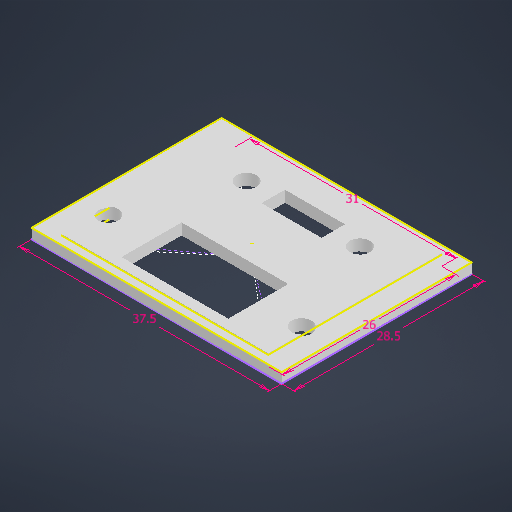
# Autodesk Inventor part: USB inner clamp plate
Saved by Autodesk Inventor 2026.2 (Build 302298010, 298A)
## iProperties
Created: 2026-04-19
Part Number: USB inner clamp plate
Material: Generic
Document SubType Name: Modeling
Designer: Graeme
Density: 1 g/cm^3
Appearance: Default
Author: Graeme
## iProperties of the stored document USB inner clamp plate_3DPrint.ipt
Created: 2026-09-30
Part Number: USB inner clamp plate_3DPrint
Material: Generic
Document SubType Name: Modeling
Designer: Graeme
Density: 1 g/cm^3
Appearance: Default
Author: Graeme
Autodesk Inventor part; units mm, degrees
ref_plane "YZ Plane" through (0, 0, 0) normal (1, 0, 0) x (0, 1, 0)
ref_plane "XZ Plane" through (0, 0, 0) normal (0, 1, 0) x (-1, 0, 0)
ref_plane "XY Plane" through (0, 0, 0) normal (0, 0, 1) x (1, 0, 0)
sketch "Sketch1" plane through (0, 0, 0) normal (0, 1, 0) x (-1, 0, 0)
  line L0 (15.5, 13) -> (-15.5, 13)
  line L1 (-15.5, 13) -> (-15.5, -13)
  line L2 (-15.5, -13) -> (15.5, -13)
  line L3 (15.5, -13) -> (15.5, 13)
  line L4 (15.5, 13) -> (-15.5, -13) construction
  line L5 (-15.5, 13) -> (15.5, -13) construction
  line L6 (18.75, -14.25) -> (-18.75, -14.25)
  line L7 (-18.75, -14.25) -> (-18.75, 14.25)
  line L8 (-18.75, 14.25) -> (18.75, 14.25)
  line L9 (18.75, 14.25) -> (18.75, -14.25)
  line L10 (18.75, -14.25) -> (-18.75, 14.25) construction
  line L11 (-18.75, -14.25) -> (18.75, 14.25) construction
  point P0 (0, 0)
  dimension "d0" = 31
  dimension "d1" = 26
  dimension "d16" = 37.5
  dimension "d17" = 28.5
  constraints: 24 end point, 4 parallel, 2 horizontal, 2 midpoint, 2 perpendicular
  measures "d0" distance of L2.end L1.end
  measures "d1" distance of L1.end L0.end
  measures "d16" distance of L7.end L8.end
  measures "d17" distance of L6.end L7.end
extrude "Extrusion2" add sketch "Sketch1" along normal blind 1.5 contours L3 L2 L1 L0 | L6 L7 L8 L9
sketch "Sketch2" plane through (0, 1.5, 0) normal (0, 1, 0) x (1, 0, 0)
  line L0 (15.5, 13) -> (-15.5, 13) projected
  line L1 (-15.5, -13) -> (15.5, -13) projected
  line L2 (-18.75, -14.25) -> (18.75, -14.25) projected
  line L3 (18.75, -14.25) -> (18.75, 14.25) projected
  line L4 (18.75, 14.25) -> (-18.75, 14.25) projected
  line L5 (-18.75, 14.25) -> (-18.75, -14.25) projected
  line L6 (15.5, -13) -> (15.5, 13) projected
  line L7 (-15.5, 13) -> (-15.5, -13) projected
  point P0 (0, 0)
extrude "Extrusion4" add sketch "Sketch2" along normal blind 0.2 contours L6 L1 L7 L0
sketch "Sketch3" plane through (0, 1.7, 0) normal (0, 1, 0) x (1, 0, 0)
  circle A0 centre (-14.5, -7) radius 1.5
  circle A1 centre (14.5, -7) radius 1.5
  circle A2 centre (-8.5, 7.75) radius 1.5
  circle A3 centre (8.5, 7.75) radius 1.5
  line L0 (0, -13.0822) -> (0, 13.0822)
  line L1 (-15.5, -13) -> (15.5, -13) projected
  line L2 (15.5, 13) -> (-15.5, 13) projected
  line L3 (8, -11.5) -> (-8, -11.5)
  line L4 (-8, -11.5) -> (-8, -2.5)
  line L5 (-8, -2.5) -> (8, -2.5)
  line L6 (8, -2.5) -> (8, -11.5)
  line L7 (8, -11.5) -> (-8, -2.5) construction
  line L8 (-8, -11.5) -> (8, -2.5) construction
  line L9 (4.5, 6) -> (-4.5, 6)
  line L10 (-4.5, 6) -> (-4.5, 9.5)
  line L11 (-4.5, 9.5) -> (4.5, 9.5)
  line L12 (4.5, 9.5) -> (4.5, 6)
  line L13 (4.5, 6) -> (-4.5, 9.5) construction
  line L14 (-4.5, 6) -> (4.5, 9.5) construction
  point P0 (0, 0)
  point P1 (0, -7)
  point P2 (0, 7.75)
  dimension "d25" = 3
  dimension "d26" = 3
  dimension "d27" = 3
  dimension "d28" = 3
  dimension "d29" = 8.5
  dimension "d30" = 8.5
  dimension "d31" = 14.5
  dimension "d32" = 14.5
  dimension "d33" = 6
  dimension "d34" = 6
  dimension "d35" = 5.25
  dimension "d36" = 5.25
  dimension "d37" = 16
  dimension "d38" = 9
  dimension "d39" = 9
  dimension "d40" = 3.5
  constraints: 26 end point, 5 midpoint, 4 centre point, 4 parallel, 2 horizontal, 2 perpendicular, 1 vertical
  measures "d25" diameter of A0
  measures "d26" diameter of A1
  measures "d27" diameter of A2
  measures "d28" diameter of A3
  measures "d29" distance from line of L0 A2.centre
  measures "d30" distance from line of L0 A3.centre
  measures "d31" distance from line of L0 A0.centre
  measures "d32" distance from line of A1.centre L0
  measures "d33" distance from line of A0.centre L1
  measures "d34" distance from line of L1 A1.centre
  measures "d35" distance from line of A2.centre L2
  measures "d36" distance from line of A3.centre L2
  measures "d37" distance of L4.end L5.end
  measures "d38" distance of L3.end L4.end
  measures "d39" distance of L10.end L11.end
  measures "d40" distance of L9.end L10.end
extrude "Extrusion5" cut sketch "Sketch3" against normal up to surface (1.7 mm away)
sketch "Sketch4" plane through (0, 0, 0) normal (0, -1, 0) x (1, 0, 0)
  line L0 (-15.5, 13) -> (15.5, 13) projected
  line L1 (15.5, 13) -> (15.5, -13) projected
  line L2 (-15.5, -13) -> (-15.5, 13) projected
  line L3 (15.5, -13) -> (-15.5, -13) projected
  point P0 (0, 0)
equation "\"d30\" = d29"
equation "\"d32\" = d31"
equation "\"d34\" = d33"
equation "\"d36\" = d35"
body "Solid2"
